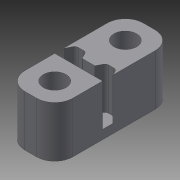
# Autodesk Inventor part: belt-clamp
Saved by Autodesk Inventor 2013 (Build 170138000, 138)
## iProperties
Created: 2013-09-28
Part Number: belt-clamp
Material: Generic
Document SubType Name: Modeling
Designer: Admin
Density: 1 g/cm^3
Author: Admin
Autodesk Inventor part; units mm, degrees
ref_plane "YZ Plane" through (0, 0, 0) normal (1, 0, 0) x (0, 1, 0)
ref_plane "XZ Plane" through (0, 0, 0) normal (0, 1, 0) x (-1, 0, 0)
ref_plane "Work Plane1" through (-367703.1992, 632830.1242, 533306.3882) normal (-0.7430322, 0.6187428, -0.2550695) x (0.5860721, 0.7855909, 0.1984099)
sketch "Sketch1" plane through (15736.2978, -8215.3634, -12939.6422) normal (-0.8717195, 0.4624093, -0.1621198) x (0.4686085, 0.883406, 0)
  circle A0 centre (-111.4493, -109512.2066) radius 1.9
  circle A1 centre (-105.9197, -109447.9073) radius 1.9
  line L0 (-1, 8.962) -> (1, 8.962)
  arc A2 (-4.0236, -0.3508) -> (-14, 8.962) centre (-14, -1.038) ccw
  arc A3 (-4, -7.838) -> (-1, -10.838) centre (-1, -7.838) ccw
  line L1 (-1, -10.838) -> (1, -10.838)
  arc A4 (1, -10.838) -> (4, -7.838) centre (1, -7.838) ccw
  line L2 (-6.0031, -0.3508) -> (-3.9739, -0.3508)
  line L3 (-421.5485, 0.712) -> (525.8715, 0.712)
  arc A5 (-3.6711, -0.5438) -> (-3.9739, -0.3508) centre (-3.9739, -0.685) ccw
  line L4 (-3.2429, -1.398) -> (-3.6711, -0.5438)
  arc A6 (-3.2429, -1.398) -> (-2.8963, -1.6208) centre (-2.8963, -1.2398) ccw
  line L5 (-2.0007, -1.6208) -> (-2.8963, -1.6208)
  arc A7 (-2.0007, -1.6208) -> (-1.6554, -1.4008) centre (-2.0007, -1.2398) ccw
  line L6 (-1.2684, -0.5708) -> (-1.6554, -1.4008)
  arc A8 (-0.9231, -0.3508) -> (-1.2684, -0.5708) centre (-0.9231, -0.7318) ccw
  line L7 (-0.9231, -0.3508) -> (1.1061, -0.3508)
  arc A9 (1.4089, -0.5438) -> (1.1061, -0.3508) centre (1.1061, -0.685) ccw
  line L8 (1.8384, -1.4008) -> (1.4089, -0.5438)
  arc A10 (1.8384, -1.4008) -> (2.1837, -1.6208) centre (2.1837, -1.2398) ccw
  line L9 (3.0793, -1.6208) -> (2.1837, -1.6208)
  arc A11 (3.0793, -1.6208) -> (3.4234, -1.4033) centre (3.0793, -1.2398) ccw
  line L10 (3.8551, -0.4948) -> (3.4234, -1.4033)
  arc A12 (4.1569, -0.304) -> (3.8551, -0.4948) centre (4.1569, -0.6382) ccw
  line L11 (4.1569, -0.304) -> (6.1861, -0.304)
  arc A13 (-1, 8.962) -> (-4, 5.962) centre (-1, 5.962) ccw
  arc A14 (4, 5.962) -> (1, 8.962) centre (1, 5.962) ccw
  line L12 (-4, -0.6008) -> (-3.9739, -0.6008)
  arc A15 (-3.8967, -0.6516) -> (-3.9739, -0.6008) centre (-3.9739, -0.685) ccw
  line L13 (-3.8967, -0.6516) -> (-3.4682, -1.5065)
  arc A16 (-3.4682, -1.5065) -> (-2.8963, -1.8708) centre (-2.8963, -1.2398) ccw
  line L14 (-2.8963, -1.8708) -> (-2.0007, -1.8708)
  arc A17 (-2.0007, -1.8708) -> (-1.4289, -1.5065) centre (-2.0007, -1.2398) ccw
  line L15 (-1.4289, -1.5065) -> (-1.0418, -0.6765)
  arc A18 (-0.9231, -0.6008) -> (-1.0418, -0.6765) centre (-0.9231, -0.7318) ccw
  line L16 (-0.9231, -0.6008) -> (1.1061, -0.6008)
  arc A19 (1.1833, -0.6516) -> (1.1061, -0.6008) centre (1.1061, -0.685) ccw
  line L17 (1.1833, -0.6516) -> (1.6135, -1.5101)
  arc A20 (1.6135, -1.5101) -> (2.1837, -1.8708) centre (2.1837, -1.2398) ccw
  line L18 (2.1837, -1.8708) -> (3.0793, -1.8708)
  arc A21 (3.0793, -1.8708) -> (3.6492, -1.5106) centre (3.0793, -1.2398) ccw
  line L19 (3.6492, -1.5106) -> (4, -0.7723)
  arc A22 (4.1569, -0.554) -> (4.0809, -0.602) centre (4.1569, -0.6382) ccw
  line L20 (4.1569, -0.554) -> (6.1861, -0.554)
  line L21 (-4, -0.6008) -> (-4, -7.838)
  line L22 (-4, 5.962) -> (-4, 0.962)
  line L23 (-4, 0.712) -> (-4, -0.3508)
  line L24 (-421.5485, 0.962) -> (-4.202, 0.962)
  line L25 (4, 0.962) -> (4, 5.962)
  arc A23 (14, 8.962) -> (4.025, -0.3311) centre (14, -1.038) ccw
  arc A24 (4.0005, -0.9335) -> (4, -1.038) centre (14, -1.038) ccw
  line L26 (4, -7.838) -> (4, -0.7723)
  line L27 (4, -0.3431) -> (4, 0.712)
  line L28 (-4, 0.962) -> (4, 0.962)
  line L29 (4.202, 0.962) -> (525.8715, 0.962)
  point P0 (-116.6614, -15646.3059)
  dimension "d0" = 3
  dimension "d2" = 3
  dimension "d3" = 0.25
  constraints: 60 end point, 51 point on circle, 25 centre point, 8 tangent, 7 point on line, 3 parallel, 1 equal radius, 13 other
  measures "d0" radius of A3
  measures "d2" radius of A13
  measures "d3" distance between parallel lines of L12 L2
extrude "Extrusion1" add sketch "Sketch1" along normal blind 7 contours L0 A14 L25 L28 L22 A13 | L21 L12 A15 L13 A16 L14 A17 L15 A18 L16 A19 L17 A20 L18 A21 L19 L26 A24 A4 L1 A3
sketch "Sketch2" plane through (15730.1957, -8212.1265, -12940.777) normal (-0.8717195, 0.4624093, -0.1621198) x (0.4686085, 0.883406, 0)
  circle A0 centre (0, 4.962) radius 1.9 projected
  line L0 (1, 8.962) -> (-1, 8.962) projected
  arc A1 (-1, 8.962) -> (-4, 5.962) centre (-1, 5.962) ccw projected
  line L1 (-4, 5.962) -> (-4, 0.962) projected
  line L2 (4, 0.962) -> (4, 5.962) projected
  arc A2 (4, 5.962) -> (1, 8.962) centre (1, 5.962) ccw projected
  circle A3 centre (0, -6.838) radius 1.9
  arc A4 (-4, -7.838) -> (-1, -10.838) centre (-1, -7.838) ccw
  line L3 (-1, -10.838) -> (1, -10.838)
  arc A5 (1, -10.838) -> (4, -7.838) centre (1, -7.838) ccw
  line L4 (4, -7.838) -> (4, -0.7723)
  line L5 (4, -0.7723) -> (4, 0.962)
  line L6 (-4, -7.838) -> (-4, 0.962)
  point P0 (-116.6614, -15646.3059)
  constraints: 8 end point, 4 point on circle, 3 centre point, 1 parallel, 1 tangent
extrude "Extrusion2" add sketch "Sketch2" along normal blind 1.5
move or copy body "Move Body1" bodies to move or copy 1 copy no rotation origin (0, 0, 0) rotation axis (-0.4686085, -0.883406, 0) rotation angle 90 translate (4249.9407, -2254.4088, -30671.5092)
move or copy body "Move Body2" bodies to move or copy 1 copy no translate (14.9738, 0, -3.187)
move or copy body "Move Body3" bodies to move or copy 1 copy no translate (0, -205.3427, 0)
move or copy body "Move Body4" bodies to move or copy 1 copy no translate (10, 0, 0)
move or copy body "Move Body5" bodies to move or copy 1 copy no translate (-10, 0, 0)
equation "\"d4\" = d3"
body "Solid1"
